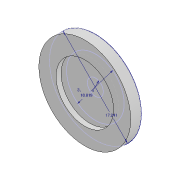
# Autodesk Inventor part: 前足中間接続スペーサ
Saved by Autodesk Inventor 2020 (Build 240168000, 168)
## iProperties
Created: 2020-11-11
Part Number: 前足中間接続スペーサ
Material: 一般
Document SubType Name: Modeling
Designer: AA19065
Density: 1 g/cm^3
Appearance: 既定
Author: AA19065
Autodesk Inventor part; units mm, degrees
ref_plane "YZ Plane" through (0, 0, 0) normal (1, 0, 0) x (0, 1, 0)
ref_plane "XZ Plane" through (0, 0, 0) normal (0, 1, 0) x (-1, 0, 0)
ref_plane "XY Plane" through (0, 0, 0) normal (0, 0, 1) x (1, 0, 0)
sketch "スケッチ1" plane through (0, 0, 0) normal (0, 0, 1) x (1, 0, 0)
  circle A0 centre (0, 0) radius 5.4095
  circle A1 centre (0, 0) radius 8.6207
  circle A2 centre (0, 0) radius 1.5
  dimension "d0" = 10.819
  dimension "d1" = 17.2414
  dimension "d6" = 3
  constraints: 3 centre point, 3 coincident
  measures "d0" diameter of A0
  measures "d1" diameter of A1
  measures "d6" diameter of A2
extrude "押し出し1" add sketch "スケッチ1" along normal blind 1 contours A0 | A2
extrude "押し出し2" add sketch "スケッチ1" along normal blind 1.95 contours A1
